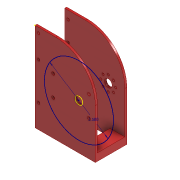
# Autodesk Inventor part: whole servo mount
Saved by Autodesk Inventor 2020 (Build 240168000, 168)
## iProperties
Created: 2019-12-15
Part Number: whole servo mount
Material: Generic
Document SubType Name: Modeling
Designer: ball
Density: 1 g/cm^3
Appearance: Default
Author: ball
Autodesk Inventor part; units mm, degrees
ref_plane "YZ Plane" through (0, 0, 0) normal (1, 0, 0) x (0, 1, 0)
ref_plane "XZ Plane" through (0, 0, 0) normal (0, 1, 0) x (-1, 0, 0)
ref_plane "XY Plane" through (0, 0, 0) normal (0, 0, 1) x (1, 0, 0)
ref_plane "Work Plane1" through (0, 0, 0) normal (0, 0, 1) x (1, 0, 0)
sketch "Sketch1" plane through (0, 0, 0) normal (0, 0, 1) x (1, 0, 0)
  line L0 (0, 0) -> (77.47, 0)
  line L1 (77.47, 0) -> (77.47, -114.3)
  line L2 (77.47, -114.3) -> (0, -114.3)
  line L3 (0, -114.3) -> (0, 0)
  circle A0 centre (56.1975, -55.5625) radius 4.8895
  circle A1 centre (4.4958, -6.5024) radius 1.7
  circle A2 centre (4.4958, -35.9918) radius 1.7
  circle A3 centre (4.4958, -83.9978) radius 1.7
  dimension "d0" = 77.47
  dimension "d1" = 114.3
  dimension "d2" = 9.779
  dimension "d42" = 3.4
  dimension "d43" = 6.5024
  dimension "d44" = 4.4958
  dimension "d53" = 3.4
  dimension "d54" = 35.9918
  dimension "d55" = 4.4958
  dimension "d56" = 3.4
  dimension "d57" = 83.9978
  dimension "d58" = 4.4958
  dimension "d64" = 56.1975
  constraints: 8 end point, 4 centre point, 2 parallel, 1 horizontal, 1 perpendicular
  measures "d0" distance of L1.end L2.end
  measures "d1" distance of L0.end L1.end
  measures "d2" diameter of A0
  measures "d42" diameter of A1
  measures "d43" distance from line of A1.centre L0
  measures "d44" distance from line of L3 A1.centre
  measures "d53" diameter of A2
  measures "d54" distance from line of L0 A2.centre
  measures "d55" distance from line of L3 A2.centre
  measures "d56" diameter of A3
  measures "d57" distance from line of L0 A3.centre
  measures "d58" distance from line of L3 A3.centre
  measures "d64" distance from line of L3 A0.centre
extrude "Servo Mount Side" add sketch "Sketch1" along normal blind 2.54
ref_plane "Work Plane2" through (0, -215, -35.5) normal (0, 0, -1) x (-1, 0, 0)
sketch "Sketch3" plane through (0, -215, -35.5) normal (0, 0, -1) x (-1, 0, 0)
  line L0 (-77.47, 215) -> (0, 215) projected
  line L1 (0, 215) -> (-77.47, 215)
  line L2 (-77.47, 215) -> (-77.47, 100.7)
  line L3 (-77.47, 100.7) -> (0, 100.7)
  line L4 (0, 100.7) -> (0, 215)
  circle A0 centre (-56.1975, 159.4375) radius 4.8895 projected
  circle A1 centre (-4.4958, 204.6622) radius 1.7
  circle A2 centre (-4.4958, 179.0082) radius 1.7
  circle A3 centre (-4.4958, 131.0022) radius 1.7
  circle A4 centre (-20, 202) radius 1.7
  dimension "d13" = 114.3
  dimension "d14" = 77.47
  dimension "d48" = 3.4
  dimension "d49" = 10.3378
  dimension "d50" = 4.4958
  dimension "d51" = 3.4
  dimension "d52" = 3.4
  dimension "d59" = 35.9918
  dimension "d60" = 83.9978
  dimension "d61" = 4.4958
  dimension "d62" = 4.4958
  dimension "d65" = 3.4
  dimension "d66" = 20
  dimension "d67" = 13
  constraints: 8 end point, 4 centre point, 2 parallel, 1 horizontal, 1 perpendicular
  measures "d13" distance between parallel lines of L0 L3
  measures "d14" distance between parallel lines of L4 L2
  measures "d48" diameter of A1
  measures "d49" distance from line of L0 A1.centre
  measures "d50" distance from line of L4 A1.centre
  measures "d51" diameter of A2
  measures "d52" diameter of A3
  measures "d59" distance from line of L0 A2.centre
  measures "d60" distance from line of L0 A3.centre
  measures "d61" distance from line of L4 A2.centre
  measures "d62" distance from line of L4 A3.centre
  measures "d65" diameter of A4
  measures "d66" distance from line of L4 A4.centre
  measures "d67" distance from line of L1 A4.centre
extrude "Encoder Mount Side" add sketch "Sketch3" along normal blind 2.54 contours L0 L4 L3 L2 | A4
sketch "Sketch4" plane through (0, -215, -35.5) normal (0, 0, 1) x (1, 0, 0)
  line L0 (77.47, 100.7) -> (0, 100.7) projected
  line L1 (10.033, 100.7) -> (29.083, 100.7)
  line L2 (29.083, 100.7) -> (29.083, 110.225)
  line L3 (29.083, 110.225) -> (10.033, 110.225)
  line L4 (10.033, 110.225) -> (10.033, 100.7)
  line L5 (77.47, 100.7) -> (58.42, 100.7)
  line L6 (58.42, 100.7) -> (58.42, 110.225)
  line L7 (58.42, 110.225) -> (77.47, 110.225)
  line L8 (77.47, 110.225) -> (77.47, 100.7)
  line L9 (0, 100.7) -> (0, 215) projected
  dimension "d20" = 19.05
  dimension "d21" = 9.525
  dimension "d22" = 19.05
  dimension "d23" = 9.525
  dimension "d63" = 10.033
  constraints: 16 end point, 4 parallel, 2 horizontal, 2 perpendicular, 1 point on line
  measures "d20" distance of L3.end L2.end
  measures "d21" distance of L2.end L1.end
  measures "d22" distance of L6.end L7.end
  measures "d23" distance of L5.end L6.end
  measures "d63" distance between parallel lines of L9 L4
extrude "Extrusion3" add sketch "Sketch4" along normal up to surface (35.5 mm away)
sketch "Sketch5" plane through (0, -215, -38.04) normal (0, 0, -1) x (-1, 0, 0)
  circle A0 centre (-65.7225, 159.4375) radius 1.397
  circle A1 centre (-56.1975, 159.4375) radius 4.8895 projected
  circle A2 centre (-62.9327, 152.7023) radius 1.397
  circle A3 centre (-56.1975, 149.9125) radius 1.397
  circle A4 centre (-49.4623, 152.7023) radius 1.397
  circle A5 centre (-46.6725, 159.4375) radius 1.397
  circle A6 centre (-49.4623, 166.1727) radius 1.397
  circle A7 centre (-56.1975, 168.9625) radius 1.397
  circle A8 centre (-62.9327, 166.1727) radius 1.397
  point P0 (0, 215)
  dimension "d26" = 2.794
  dimension "d27" = 9.525
  dimension "d30" = 360
  constraints: 8 centre point, 17 other
  measures "d26" diameter of A0
  measures "d27" distance of A1.centre A0.centre
extrude "Extrusion4" cut sketch "Sketch5" against normal blind 2.54
sketch "Sketch7" plane through (0, 0, 0) normal (0, 0, -1) x (-1, 0, 0)
  circle A0 centre (-49.4623, -62.2977) radius 1.397 projected
  circle A1 centre (-49.4623, -48.8273) radius 1.397 projected
  circle A2 centre (-65.7225, -55.5625) radius 1.397 projected
  circle A3 centre (-46.6725, -55.5625) radius 1.397 projected
  circle A4 centre (-62.9327, -48.8273) radius 1.397 projected
  circle A5 centre (-62.9327, -62.2977) radius 1.397 projected
  circle A6 centre (-56.1975, -65.0875) radius 1.397 projected
  circle A7 centre (-56.1975, -46.0375) radius 1.397 projected
  line L0 (0, -114.3) -> (0, 0) projected
  line L1 (0, 0) -> (-77.47, 0) projected
  line L2 (-77.47, 0) -> (-77.47, -114.3) projected
  line L3 (-77.47, -114.3) -> (0, -114.3) projected
  circle A8 centre (-56.1975, -55.5625) radius 4.8895 projected
  circle A9 centre (-69.3421, -42.0921) radius 1.3525 construction
  circle A10 centre (-23.3529, -42.0921) radius 1.3525 construction
  circle A11 centre (-23.3529, -69.0329) radius 1.3525 construction
  circle A12 centre (-69.3421, -69.0329) radius 1.3525 construction
  circle A13 centre (-69.3421, -69.0329) radius 1.9304
  circle A14 centre (-69.3421, -42.0921) radius 1.9304
  circle A15 centre (-23.3529, -42.0921) radius 1.9304
  circle A16 centre (-23.3529, -69.0329) radius 1.9304
  point P0 (0, 0)
  dimension "d34" = 3.8608
  dimension "d35" = 3.8608
  dimension "d36" = 3.8608
  dimension "d37" = 3.8608
  constraints: 4 centre point, 4 coincident
  measures "d34" diameter of A13
  measures "d35" diameter of A14
  measures "d36" diameter of A15
  measures "d37" diameter of A16
extrude "Extrusion5" cut sketch "Sketch7" against normal through all contours A13 | A14 | A15 | A16
sketch "Sketch8" plane through (0, 0, 2.54) normal (0, 0, 1) x (1, 0, 0)
  circle A0 centre (56.1975, -55.5625) radius 4.8895 projected
  circle A1 centre (56.1975, -55.5625) radius 44.45
  point P0 (0, 0)
  dimension "d40" = 88.9
  constraints: 1 centre point, 1 coincident
  measures "d40" diameter of A1
fillet "Fillet1" radius 50.8 2 edges at (77.47, 0, -36.77) (77.47, 0, 1.27)
equation "\"d55\" = d44"
equation "\"d58\" = d44"
equation "\"d13\" = d1"
equation "\"d14\" = d0"
equation "\"d50\" = d44"
equation "\"d61\" = d44"
equation "\"d62\" = d44"
body "Solid1"
